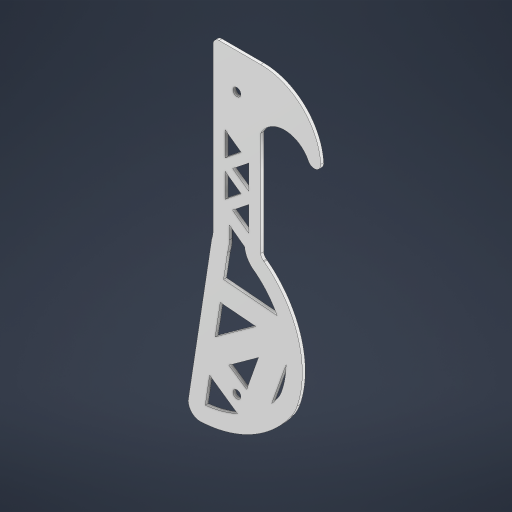
# Autodesk Inventor part: sled
Saved by Autodesk Inventor 2024 (Build 280153000, 153)
## iProperties
Created: 2023-10-27
Part Number: sled
Material: Acetal Resin, White
Document SubType Name: Sheet Metal
Designer: Averey Ku
Density: 1.425 g/cm^3
Appearance: Smooth - White
Flat Pattern Width: 7.067 cm
Flat Pattern Length: 18.1066 cm
Flat Pattern Area: 127.959 cm^2
Sheet Metal Rule: Default
Sheet Metal Width: 2.782 in
Sheet Metal Length: 7.129 in
Sheet Metal Area: 19.834 in^2
Author: Averey Ku
Autodesk Inventor part; units mm, degrees
ref_plane "YZ Plane" through (0, 0, 0) normal (1, 0, 0) x (0, 1, 0)
ref_plane "XZ Plane" through (0, 0, 0) normal (0, 1, 0) x (-1, 0, 0)
ref_plane "XY Plane" through (0, 0, 0) normal (0, 0, 1) x (1, 0, 0)
sketch "Sketch1" plane through (0, 0, 0) normal (0, 0, 1) x (1, 0, 0)
  circle A0 centre (-26.9881, -17.2743) radius 2.0955
  circle A1 centre (-26.9881, 46.2257) radius 2.0955
  arc A2 (-46.2652, -39.5915) -> (1.8146, -13.1917) centre (-49.3718, 23.0479) ccw
  arc A3 (5.1303, -6.697) -> (-12.4868, 51.2687) centre (-44.0163, 10.0263) ccw
  line L0 (-52.8546, -32.2756) -> (-40.5161, 47.238)
  arc A4 (1.8146, -13.1917) -> (5.1303, -6.697) centre (-18.9158, 1.4852) ccw
  arc A5 (-52.8546, -32.2756) -> (-46.2652, -39.5915) centre (-46.5797, -33.2493) ccw
  arc A6 (-40.2918, 48.1911) -> (-40.5161, 47.238) centre (-34.2412, 46.2643) ccw
  arc A7 (-12.4868, 51.2687) -> (-12.8478, 51.5252) centre (-16.3434, 46.224) ccw
  circle A8 centre (-26.9881, 122.4257) radius 2.0955
  line L1 (-14.2749, 54.1759) -> (-14.2749, 109.7164)
  line L2 (-39.693, 122.4164) -> (-39.693, 52.0448)
  arc A9 (11.1869, 109.6057) -> (-14.2749, 109.7164) centre (-1.5714, 103.3543) ccw
  arc A10 (11.1869, 109.6057) -> (17.7339, 111.3354) centre (14.2875, 111.125) ccw
  arc A11 (-14.2749, 128.7664) -> (-14.293, 128.7664) centre (-14.293, 89.434) ccw
  arc A12 (-40.2918, 48.1911) -> (-39.693, 52.0448) centre (-52.393, 52.0448) ccw
  arc A13 (-14.2749, 54.1759) -> (-12.8478, 51.5252) centre (-11.0999, 54.1759) ccw
  line L3 (-14.293, 141.4664) -> (-36.518, 141.4664)
  line L4 (-39.693, 138.2914) -> (-39.693, 122.4164)
  arc A14 (17.7339, 111.3354) -> (-14.293, 141.4664) centre (-14.293, 109.3798) ccw
  arc A15 (-36.518, 141.4664) -> (-39.693, 138.2914) centre (-36.518, 138.2914) ccw
  line L5 (-20.6375, 60.325) -> (-29.3177, 66.7014)
  line L6 (-29.3177, 66.7014) -> (-20.6375, 73.6265)
  line L7 (-33.3304, 69.6491) -> (-24.7096, 76.5269)
  line L8 (-24.7096, 76.5269) -> (-33.3304, 82.6673)
  line L9 (-20.6375, 79.7757) -> (-29.2584, 85.916)
  line L10 (-29.2584, 85.916) -> (-20.6375, 92.7938)
  line L11 (-33.3304, 88.8164) -> (-24.7096, 95.6942)
  line L12 (-24.7096, 95.6942) -> (-33.3304, 101.8346)
  line L13 (-20.6375, 98.943) -> (-29.121, 104.9855)
  line L14 (-29.121, 104.9855) -> (-20.6375, 111.3354)
  line L15 (-20.6375, 73.6265) -> (-20.6375, 60.325)
  line L16 (-33.3304, 69.6491) -> (-33.3304, 82.6673)
  line L17 (-20.6375, 111.0754) -> (-20.6375, 98.943)
  line L18 (-20.6375, 92.7938) -> (-20.6375, 79.7757)
  line L19 (-33.3304, 88.8164) -> (-33.3304, 101.8346)
  line L20 (-35.8728, 20.7599) -> (-16.8764, 19.1555)
  line L21 (-16.8764, 19.1555) -> (-38.5549, 3.4753)
  line L22 (-38.5549, 3.4753) -> (-35.8728, 20.7599)
  line L23 (-15.465, 5.4956) -> (-31.2539, -5.9246)
  line L24 (-31.2539, -5.9246) -> (-21.7628, -12.4092)
  line L25 (-21.7628, -12.4092) -> (-15.465, 5.4956)
  line L26 (-26.6964, -26.0353) -> (-41.5352, -15.7309)
  line L27 (-41.5352, -15.7309) -> (-43.8641, -30.7387)
  arc A16 (-43.8641, -30.7387) -> (-26.6964, -26.0353) centre (-49.3718, 23.0479) ccw
  line L28 (-0.7544, 9.4821) -> (-8.3865, -12.216)
  arc A17 (-8.3865, -12.216) -> (-5.244, -8.1943) centre (-49.3718, 23.0479) ccw
  arc A18 (-5.244, -8.1943) -> (-3.0573, -3.911) centre (-18.9158, 1.4852) ccw
  arc A19 (-3.0573, -3.911) -> (-0.7544, 9.4821) centre (-44.0163, 10.0263) ccw
  arc A20 (-22.8622, 52.9736) -> (-17.68, 44.3525) centre (-11.0999, 54.1759) ccw
  line L29 (-22.8622, 52.9736) -> (-31.0444, 58.9842)
  line L30 (-31.0444, 58.9842) -> (-31.0444, 52.0448)
  arc A21 (-31.9963, 45.7412) -> (-31.0444, 52.0448) centre (-52.393, 52.0448) ccw
  line L31 (-31.9963, 45.7412) -> (-34.0923, 32.2341)
  line L32 (-34.0923, 32.2341) -> (-5.5459, 29.8231)
  arc A22 (-5.5459, 29.8231) -> (-17.68, 44.3525) centre (-44.0163, 10.0263) ccw
  point P0 (-53.9756, -39.4993)
  point P1 (-26.9881, 52.574)
  point P2 (-14.2749, 52.2277)
  point P3 (-39.693, 128.7664)
  point P4 (-39.693, 49.5201)
  dimension "d5" = 4.191
  dimension "d6" = 4.191
  dimension "d7" = 25.4
  dimension "d8" = 6.35
  dimension "d9" = 6.35
  dimension "d11" = 4.191
  dimension "d13" = 25.4
  dimension "d15" = 19.05
  dimension "d18" = 12.7
  dimension "d19" = 3.175
  dimension "d20" = 12.7
  dimension "d21" = 3.175
  constraints: 66 end point, 43 point on circle, 23 centre point, 16 tangent, 6 parallel, 5 point on line, 1 equal radius, 1 horizontal, 1 perpendicular, 1 vertical, 4 other
  measures "d5" diameter of A0
  measures "d6" diameter of A1
  measures "d7" radius of A4
  measures "d8" radius of A5
  measures "d9" radius of A6
  measures "d11" diameter of A8
  measures "d13" distance of A11.end point (-39.693, 128.766)
  measures "d15" distance of L1.end A11.end
  measures "d18" radius of A12
  measures "d19" radius of A13
  measures "d20" distance of A11.end L3.start
  measures "d21" radius of A15
extrude "Extrusion1" add sketch "Sketch1" along normal blind 1.5875 contours A5 L0 A6 A12 L2 L4 A15 L3 A14 A10 A9 L1 A13 A7 A3 A4 A2
equation "\"BendRadius\" = Thickness"
equation "\"BendReliefWidth\" = Thickness"
equation "\"BendReliefDepth\" = 0.5 * Thickness"
equation "\"CornerReliefSize\" = 4 * Thickness"
equation "\"MinimumRemnant\" = 2 * Thickness"
equation "\"TransitionRadius\" = BendRadius"
equation "\"JacobiRadiusSize\" = BendRadius"
equation "\"GapSize\" = Thickness"
equation "\"Thickness\" = 1.5875"
body "Solid1"
